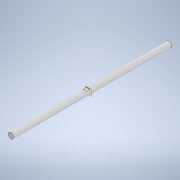
# Autodesk Inventor part: Eje_Engranes_llanta
Saved by Autodesk Inventor 2021 (Build 250183000, 183)
## iProperties
Created: 2021-02-06
Part Number: Eje_Engranes_llanta
Material: Genérico
Document SubType Name: Modeling
Designer: rotje
Density: 1 g/cm^3
Appearance: Valor por defecto
Author: rotje
Autodesk Inventor part; units mm, degrees
ref_plane "YZ Plane" through (0, 0, 0) normal (1, 0, 0) x (0, 1, 0)
ref_plane "XZ Plane" through (0, 0, 0) normal (0, 1, 0) x (-1, 0, 0)
sketch "Boceto1" plane through (0, 0, 0) normal (0, 0, 1) x (1, 0, 0)
  circle A0 centre (0, 0) radius 7.5
  dimension "d0" = 15
  constraints: 1 centre point, 1 coincident
  measures "d0" diameter of A0
extrude "Extrusión1" add sketch "Boceto1" along normal mid plane 420
ref_plane "Plano de trabajo1" through (0, 0, 5) normal (0, 0, 1) x (1, 0, 0)
sketch "Boceto5" plane through (0, 0, 5) normal (0, 0, 1) x (1, 0, 0)
  circle A0 centre (0, 0) radius 7.5
  circle A1 centre (0, 0) radius 7.5 projected
  line L0 (0, 0) -> (0, 7.5)
  line L1 (0, 7.5) -> (0, 6)
  line L2 (0, 6) -> (4.5, 6)
  arc A2 (4.5, 6) -> (-4.5, 6) centre (0, 0) ccw
  line L3 (0, 6) -> (-4.5, 6)
  point P0 (-4.5, 6)
  dimension "d10" = 15
  dimension "d11" = 1.5
  constraints: 8 end point, 5 point on circle, 1 centre point, 1 coincident, 1 horizontal, 1 perpendicular, 1 point on line, 1 vertical, 3 other
  measures "d11" distance of L0.end L1.end
extrude "Extrusión4" cut sketch "Boceto5" along normal blind 10 contours L2 L0 A0 | A0 L0 L3
